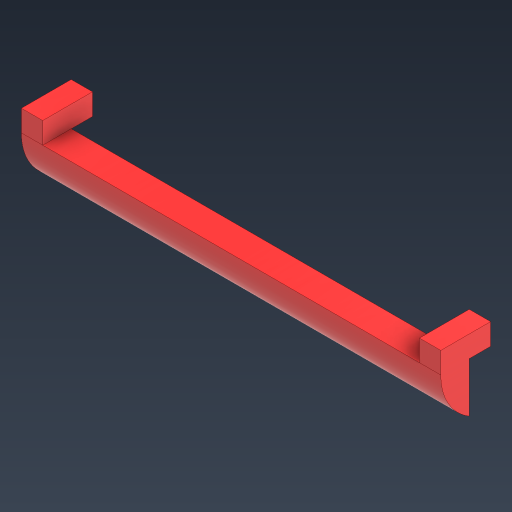
# Autodesk Inventor part: Нижний край
Saved by Autodesk Inventor 2023.2 (Build 272271030, 271C)
## iProperties
Created: 2025-08-19
Part Number: Нижний край
Material: Типовые
Document SubType Name: Modeling
Designer: Олег Коноваленко
Density: 1 g/cm^3
Appearance: Светло-красный
Author: Олег Коноваленко
Autodesk Inventor part; units mm, degrees
ref_plane "YZ Plane" through (0, 0, 0) normal (1, 0, 0) x (0, 1, 0)
ref_plane "XZ Plane" through (0, 0, 0) normal (0, 1, 0) x (-1, 0, 0)
ref_plane "XY Plane" through (0, 0, 0) normal (0, 0, 1) x (1, 0, 0)
sketch "Эскиз1" plane through (0, 0, 0) normal (1, 0, 0) x (0, 1, 0)
  line L0 (20.1556, 25.3526) -> (20.1556, -14.6474)
  line L1 (20.1556, -14.6474) -> (-49.8444, -14.6474)
  arc A0 (20.1556, 25.3526) -> (-49.8444, -14.6474) centre (20.1556, -55.8974) ccw
  line L2 (20.1556, -14.6474) -> (-20.1556, 14.6474) construction
  point P0 (0, 0)
  point P1 (0, 0)
  dimension "d0" = 70
  dimension "d2" = 40
  constraints: 6 end point, 3 point on circle, 1 centre point, 1 coincident, 1 line through centre, 1 midpoint, 1 perpendicular, 1 vertical
  measures "d0" distance of L0.end L1.end
  measures "d2" distance of L0.start L0.end
extrude "Выдавливание1" add sketch "Эскиз1" along normal mid plane 590
sketch "Эскиз6" plane through (295, 0, 0) normal (1, 0, 0) x (0, 0, -1)
  line L0 (14.6474, 20.1556) -> (-25.3526, 20.1556) projected
  line L1 (-25.3526, 20.1556) -> (44.6474, 20.1556)
  line L2 (44.6474, 20.1556) -> (44.6474, 50.1556)
  line L3 (44.6474, 50.1556) -> (-25.3526, 50.1556)
  line L4 (-25.3526, 50.1556) -> (-25.3526, 20.1556)
  point P0 (0, 0)
  dimension "d13" = 70
  dimension "d14" = 30
  constraints: 8 end point, 2 parallel, 1 horizontal, 1 perpendicular
  measures "d13" distance of L2.end L3.end
  measures "d14" distance of L3.end L0.end
extrude "Выдавливание3" add sketch "Эскиз6" against normal blind 30
mirror "Зеркальное отражение3" about plane through (0, 0, 0) normal (1, 0, 0) of "Выдавливание3"
